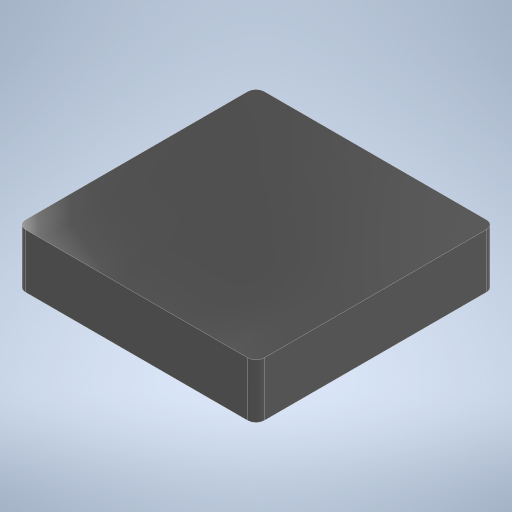
# Autodesk Inventor part: Cap
Saved by Autodesk Inventor 2023 (Build 270158000, 158)
## iProperties
Created: 2022-09-20
Part Number: Cap
Material: Стекло, литое, серое
Document SubType Name: Modeling
Designer: Makar
Density: 2.3 g/cm^3
Appearance: Темно-серый
Mass: 42.3592 g
Surface Area: 67.8991 cm^2
Volume: 18.4171 cm^3
Author: Makar
Autodesk Inventor part; units mm, degrees
ref_plane "YZ Plane" through (0, 0, 0) normal (1, 0, 0) x (0, 1, 0)
ref_plane "XZ Plane" through (0, 0, 0) normal (0, 1, 0) x (-1, 0, 0)
ref_plane "XY Plane" through (0, 0, 0) normal (0, 0, 1) x (1, 0, 0)
sketch "Эскиз1" plane through (0, 0, 0) normal (0, 1, 0) x (-1, 0, 0)
  arc A0 (41, -50) -> (45.5, -45.5) centre (41, -45.5) ccw
  line L0 (0, -50) -> (41, -50)
  arc A1 (-4.5, -45.5) -> (0, -50) centre (0, -45.5) ccw
  line L1 (-4.5, -4.5) -> (-4.5, -45.5)
  arc A2 (0, 0) -> (-4.5, -4.5) centre (0, -4.5) ccw
  line L2 (-1.5, -45.5) -> (-1.5, -4.5)
  arc A3 (0, -3) -> (-1.5, -4.5) centre (0, -4.5) ccw
  line L3 (0, -3) -> (41, -3)
  line L4 (41, 0) -> (0, 0)
  arc A4 (45.5, -4.5) -> (41, 0) centre (41, -4.5) ccw
  line L5 (45.5, -45.5) -> (45.5, -4.5)
  line L6 (42.5, -4.5) -> (42.5, -45.5)
  arc A5 (42.5, -4.5) -> (41, -3) centre (41, -4.5) ccw
  line L7 (41, -47) -> (0, -47)
  arc A6 (41, -47) -> (42.5, -45.5) centre (41, -45.5) ccw
  arc A7 (-1.5, -45.5) -> (0, -47) centre (0, -45.5) ccw
  circle A8 centre (20.5, -25) radius 18.5
  circle A9 centre (20.5, -25) radius 16.5
  circle A10 centre (20.5, -25) radius 14.5
  circle A11 centre (20.5, -25) radius 13.5
  point P0 (11.5, -30)
  constraints: 16 end point, 16 point on circle, 12 centre point
extrude "Выдавливание1" add sketch "Эскиз1" along normal blind 10 contours L2 A3 L3 A5 L6 A6 L7 A7 | A8 | A9 | A10 | A11
extrude "Выдавливание2" cut sketch "Эскиз1" along normal blind 3 contours A8 | A10
